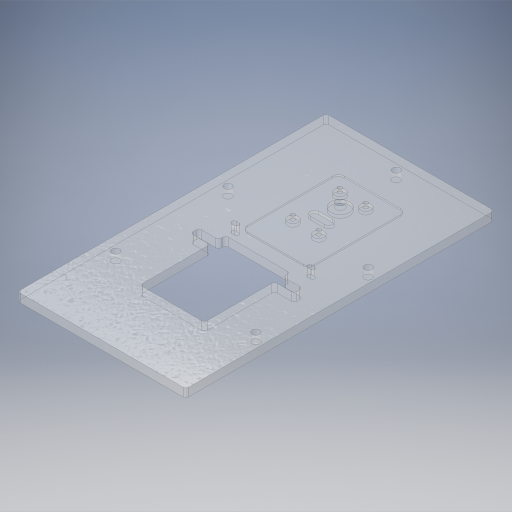
# Autodesk Inventor part: getriebe_platte_0
Saved by Autodesk Inventor 2023 (Build 270158000, 158)
## iProperties
Company: HTBLA Kaindorf
RuleStatus: InUse
Created: 2022-08-03
Part Number: getriebe_platte_0
Project: Zeichenmaschine_v2
Material: Acryl
Description: Platte Getriebemotor
Document SubType Name: Modeling
Designer: trajan20
Density: 1.188 g/cm^3
Appearance: Transparent - farblos
Mass: 160.681 g
Surface Area: 535.055 cm^2
Volume: 135.253 cm^3
AfterDocNew0: iProperties-Editor_aufrufen
Author: jan
Keywords: 2021
Autodesk Inventor part; units mm, degrees
ref_plane "YZ Plane" through (0, 0, 0) normal (1, 0, 0) x (0, 1, 0)
ref_plane "XZ Plane" through (0, 0, 0) normal (0, 1, 0) x (-1, 0, 0)
derived "BT000_trajan20_22_Zeichenmaschine_neu_Masterskizze.ipt"
sketch "Skizze3" plane through (0, 0, 0) normal (0, 0, 1) x (1, 0, 0)
  line L0 (0, 0) -> (-110, 0)
  line L1 (-220, 0) -> (-220, 120)
  line L2 (-220, 120) -> (0, 120)
  line L3 (0, 120) -> (0, 0)
  line L4 (-248.2253, 60) -> (-229.9902, 60) construction
  line L5 (-110, -37.5982) -> (-110, -22.8575) construction
  line L6 (-110, 0) -> (-220, 0)
  point P0 (-220, 60)
  point P1 (-110, 120)
  point P2 (-165, 0)
  point P3 (-60, 10)
  point P4 (-140, 10)
  point P5 (-140, 110)
  point P6 (-60, 110)
  point P7 (-60, 10)
  point P8 (-210, 60)
  dimension "d4" = 120
  dimension "d5" = 220
  dimension "d40" = 10
  dimension "d41" = 10
  dimension "d42" = 10
  dimension "d43" = 10
  dimension "d51" = 80
  dimension "d52" = 80
  dimension "d64" = 60
  dimension "d142" = 10
  dimension "d143" = 60
  constraints: 14 end point, 3 horizontal, 3 midpoint, 3 parallel, 3 point on line, 2 perpendicular, 1 coincident, 1 vertical, 1 vertical alignment
  measures "d4" distance between parallel lines of L0 L2
  measures "d5" distance between parallel lines of L1 L3
  measures "d40" distance from line of L2 point (-60, 110)
  measures "d41" distance from line of L0 point (-60, 10)
  measures "d42" distance from line of L6 point (-140, 10)
  measures "d43" distance from line of L2 point (-140, 110)
  measures "d51" distance from line of L1 point (-140, 10)
  measures "d52" distance from line of L1 point (-140, 110)
  measures "d64" distance from line of L3 point (-60, 10)
  measures "d142" distance from line of L1 point (-210, 60)
  measures "d143" distance from line of L6 point (-210, 60)
extrude "Extrusion3" add sketch "Skizze3" against normal blind 6
fillet "Rundung1" radius 2 4 edges at (-220, 120, -3) (-220, 0, -3) (0, 120, -3) (0, 0, -3)
hole "Bohrung2" at (-60, 10, 0) at (-140, 10, 0) at (-140, 110, 0) at (-60, 110, 0) at (-210, 60, 0) direction (0, 0, -1) diameter 5.5 end through all
derived "Getriebemotor.ipt"
ref_plane "Arbeitsebene3" through (0, 0, -4) normal (0, 0, -1) x (-1, 0, 0)
sketch "Skizze5" plane through (0, 0, -4) normal (0, 0, -1) x (-1, 0, 0)
  line L0 (138.8, 44) -> (138.8, 76)
  circle A0 centre (179.05, 69.25) radius 1.55
  circle A1 centre (179.05, 69.25) radius 3.775
  circle A2 centre (145.55, 69.25) radius 3.775
  circle A3 centre (145.55, 69.25) radius 1.55
  circle A4 centre (145.55, 50.75) radius 3.775
  circle A5 centre (145.55, 50.75) radius 1.55
  circle A6 centre (170, 60) radius 3.1
  circle A7 centre (170, 60) radius 6.675
  line L1 (184.8, 76) -> (184.8, 44)
  line L2 (184.8, 44) -> (138.8, 44)
  line L3 (138.8, 76) -> (184.8, 76)
  circle A8 centre (179.05, 50.75) radius 1.55
  circle A9 centre (179.05, 50.75) radius 3.775
  line L4 (220, 2) -> (220, 118) projected
  line L5 (218, 120) -> (2, 120) projected
  line L6 (0, 118) -> (0, 2) projected
  line L7 (156.8, 65) -> (156.8, 55) construction
  line L8 (153.7, 65) -> (153.7, 55)
  line L9 (159.9, 55) -> (159.9, 65)
  arc A10 (159.9, 65) -> (153.7, 65) centre (156.8, 65) ccw
  arc A11 (153.7, 55) -> (159.9, 55) centre (156.8, 55) ccw
  point P0 (0, 0)
  point P1 (184.8, 60)
  point P2 (220, 60)
  point P3 (138.8, 60)
  point P4 (0, 60)
  point P5 (156.8, 60)
  dimension "d112" = 6.75
  dimension "d113" = 6.75
  dimension "d114" = 6.75
  dimension "d115" = 6.75
  dimension "d116" = 32
  dimension "d117" = 46
  dimension "d124" = 3.1
  dimension "d125" = 3.1
  dimension "d126" = 7.55
  dimension "d127" = 16
  dimension "d128" = 14.8
  dimension "d129" = 5.75
  dimension "d131" = 5.75
  dimension "d132" = 6.75
  dimension "d133" = 6.75
  dimension "d135" = 13.35
  dimension "d136" = 3.1
  dimension "d137" = 7.55
  dimension "d138" = 7.55
  dimension "d139" = 3.1
  dimension "d140" = 50
  dimension "d242" = 6.2
  dimension "d243" = 18
  dimension "d244" = 10
  dimension "d245" = 6.2
  constraints: 16 end point, 12 centre point, 5 concentric, 5 midpoint, 5 parallel, 4 point on circle, 4 tangent, 3 horizontal alignment, 1 equal radius, 1 vertical
  measures "d112" distance from line of L2 A4.centre
  measures "d113" distance from line of L0 A4.centre
  measures "d114" distance from line of L0 A3.centre
  measures "d115" distance from line of L3 A3.centre
  measures "d116" distance of L0.start L0.end
  measures "d117" distance of L1.end L0.start
  measures "d124" diameter of A5
  measures "d125" diameter of A3
  measures "d126" diameter of A2
  measures "d127" distance from line of L2 A7.centre
  measures "d128" distance from line of L1 A7.centre
  measures "d129" distance from line of L1 A1.centre
  measures "d131" distance from line of L1 A8.centre
  measures "d132" distance from line of L2 A8.centre
  measures "d133" distance from line of L3 A0.centre
  measures "d135" diameter of A7
  measures "d136" diameter of A8
  measures "d137" diameter of A9
  measures "d138" diameter of A1
  measures "d139" diameter of A0
  measures "d140" distance from line of L4 A6.centre
  measures "d242" diameter of A6
  measures "d243" distance from line of L0 point (156.8, 60)
  measures "d244" distance of L7.start L7.end
  measures "d245" distance between parallel lines of L8 L9
sketch "Skizze6" plane through (0, 0, -6) normal (0, 0, -1) x (-1, 0, 0)
  circle A0 centre (60, 110) radius 2.75 projected
  circle A1 centre (140, 10) radius 2.75 projected
  circle A2 centre (60, 10) radius 2.75 projected
  circle A3 centre (140, 110) radius 2.75 projected
  circle A4 centre (210, 60) radius 2.75 projected
  arc A5 (0, 2) -> (2, 0) centre (2, 2) ccw projected
  line L0 (2, 0) -> (218, 0) projected
  arc A6 (218, 0) -> (220, 2) centre (218, 2) ccw projected
  line L1 (220, 2) -> (220, 118) projected
  arc A7 (220, 118) -> (218, 120) centre (218, 118) ccw projected
  line L2 (218, 120) -> (2, 120) projected
  arc A8 (2, 120) -> (0, 118) centre (2, 118) ccw projected
  line L3 (0, 118) -> (0, 2) projected
  circle A9 centre (179.05, 69.25) radius 3.775 projected
  line L4 (138.8, 76) -> (184.8, 76) projected
  line L5 (184.8, 76) -> (184.8, 44) projected
  circle A10 centre (179.05, 50.75) radius 3.775 projected
  circle A11 centre (179.05, 50.75) radius 1.55 projected
  line L6 (184.8, 44) -> (138.8, 44) projected
  line L7 (138.8, 44) -> (138.8, 76) projected
  circle A12 centre (145.55, 50.75) radius 3.775 projected
  circle A13 centre (145.55, 50.75) radius 1.55 projected
  circle A14 centre (145.55, 69.25) radius 3.775 projected
  circle A15 centre (145.55, 69.25) radius 1.55 projected
  circle A16 centre (170, 60) radius 6.675 projected
  circle A17 centre (170, 60) radius 3.1 projected
  circle A18 centre (179.05, 69.25) radius 1.55 projected
  line L8 (123.8, 84) -> (192.8, 84)
  line L9 (192.8, 84) -> (192.8, 36)
  line L10 (192.8, 36) -> (123.8, 36)
  line L11 (123.8, 36) -> (123.8, 84)
  line L12 (138.8, 62.5) -> (103.8, 62.5)
  line L13 (138.8, 57.5) -> (103.8, 57.5)
  line L14 (103.8, 67.5) -> (138.8, 67.5)
  line L15 (138.8, 57.5) -> (103.8, 67.5) construction
  line L16 (103.8, 57.5) -> (138.8, 67.5) construction
  line L17 (97.7, 99.5) -> (103.8, 99.5)
  line L18 (97.7, 25.5) -> (97.7, 99.5)
  line L19 (97.7, 85.5) -> (47.7, 85.5)
  line L20 (47.7, 39.5) -> (97.7, 39.5)
  line L21 (103.8, 99.5) -> (103.8, 25.5)
  line L22 (103.8, 25.5) -> (97.7, 25.5)
  line L23 (47.7, 39.5) -> (47.7, 85.5)
  line L24 (119.8, 90.5) -> (119.8, 88.5) construction
  line L25 (118.2, 90.5) -> (118.2, 88.5)
  line L26 (121.4, 88.5) -> (121.4, 90.5)
  arc A19 (121.4, 90.5) -> (118.2, 90.5) centre (119.8, 90.5) ccw
  arc A20 (118.2, 88.5) -> (121.4, 88.5) centre (119.8, 88.5) ccw
  line L27 (119.8, 36.5) -> (119.8, 34.5) construction
  line L28 (118.2, 36.5) -> (118.2, 34.5)
  line L29 (121.4, 34.5) -> (121.4, 36.5)
  arc A21 (121.4, 36.5) -> (118.2, 36.5) centre (119.8, 36.5) ccw
  arc A22 (118.2, 34.5) -> (121.4, 34.5) centre (119.8, 34.5) ccw
  line L30 (103.8, 39.5) -> (108.8, 39.5)
  line L31 (108.8, 39.5) -> (108.8, 85.5)
  line L32 (108.8, 85.5) -> (95.8, 85.5)
  line L33 (159.9, 55) -> (159.9, 65) projected
  line L34 (153.7, 65) -> (153.7, 55) projected
  arc A23 (159.9, 65) -> (153.7, 65) centre (156.8, 65) ccw projected
  arc A24 (153.7, 55) -> (159.9, 55) centre (156.8, 55) ccw projected
  point P0 (0, 0)
  point P1 (138.8, 60)
  point P2 (123.8, 60)
  point P3 (121.3, 62.5)
  point P4 (138.8, 67.5)
  point P5 (138.8, 57.5)
  point P6 (92.3, 62.6)
  point P7 (95.8, 62.6)
  point P8 (97.7, 62.5)
  point P9 (97.7, 39.5)
  point P10 (47.7, 62.5)
  point P11 (119.8, 89.5)
  point P12 (119.8, 35.5)
  point P13 (100.75, 25.5)
  point P14 (108.8, 67.5)
  point P15 (102.3, 85.5)
  point P16 (103.8, 85.5)
  dimension "d158" = 8
  dimension "d159" = 8
  dimension "d160" = 15
  dimension "d161" = 8
  dimension "d165" = 10
  dimension "d170" = 6.1
  dimension "d174" = 50
  dimension "d175" = 46
  dimension "d191" = 23
  dimension "d220" = 50
  dimension "d225" = 16
  dimension "d226" = 16
  dimension "d227" = 10
  dimension "d228" = 10
  dimension "d229" = 2
  dimension "d230" = 2
  dimension "d231" = 1.6
  dimension "d232" = 1.6
  dimension "d235" = 74
  dimension "d236" = 5
  dimension "d237" = 46
  dimension "d265" = 18.5
  dimension "d266" = 35
  dimension "d267" = 5
  constraints: 54 end point, 12 midpoint, 8 parallel, 8 point on circle, 8 tangent, 6 horizontal, 4 centre point, 4 point on line, 4 vertical, 3 perpendicular, 1 horizontal alignment
  measures "d158" distance between parallel lines of L4 L8
  measures "d159" distance between parallel lines of L6 L10
  measures "d160" distance of point (138.8, 60) point (123.8, 60)
  measures "d161" distance between parallel lines of L5 L9
  measures "d165" distance of L13.end L14.start
  measures "d170" distance of L17.start L17.end
  measures "d174" distance of L20.start L20.end
  measures "d175" distance of L19.end L20.start
  measures "d191" distance between parallel lines of L19 L12
  measures "d220" distance from line of L18 point (47.7, 62.5)
  measures "d225" distance from line of point (119.8, 35.5) L21
  measures "d226" distance from line of L21 point (119.8, 89.5)
  measures "d227" vertical distance of point (119.8, 35.5) point (100.75, 25.5)
  measures "d228" vertical distance of L17.end point (119.8, 89.5)
  measures "d229" distance of L27.start L27.end
  measures "d230" distance of L24.start L24.end
  measures "d231" radius of A19
  measures "d232" radius of A22
  measures "d235" distance from line of L21.end L17
  measures "d236" distance of L30.start L30.end
  measures "d237" distance of L30.end L31.end
  measures "d265" distance between parallel lines of L6 L12
  measures "d266" distance between parallel lines of L7 L21
  measures "d267" distance between parallel lines of L12 L13
extrude "Extrusion10" cut sketch "Skizze6" against normal blind 1 contours L7 L14 L11 L8 L9 L10 L13 L6 L5 L4 | L4 L5 L6 L7 | L7 L12 L11 L14 | L7 L13 L11 L12 | A24 L34 A23 L33
extrude "Extrusion11" cut sketch "Skizze6" against normal blind 3.2 contours A9 | A10 | A12 | A14 | A16 | A18 | A24 L34 A23 L33
extrude "Extrusion12" cut sketch "Skizze6" against normal blind 8 contours A11 | A13 | A15 | A17 | A18
fillet "Rundung3" radius 4 4 edges at (-123.8, 84, -5.5) (-192.8, 84, -5.5) (-192.8, 36, -5.5) (-123.8, 36, -5.5)
extrude "Extrusion13" cut sketch "Skizze6" against normal blind 8 contours L21 L22 L18 L32 | L32 L18 L17 L21 | L18 L20 L23 L19
fillet "Rundung4" radius 2 8 edges at (-97.7, 99.5, -3) (-103.8, 99.5, -3) (-97.7, 25.5, -3) (-97.7, 39.5, -3) (-97.7, 85.5, -3) (-47.7, 39.5, -3) (-47.7, 85.5, -3) (-103.8, 25.5, -3)
extrude "Extrusion14" cut sketch "Skizze6" against normal blind 8 contours A19 L26 A20 L25 | A21 L29 A22 L28
extrude "Extrusion15" cut sketch "Skizze6" against normal blind 10 contours L31 L12 L21 L14 | L14 L21 L32 L31 | L31 L13 L21 L12 | L31 L30 L21 L13
fillet "Rundung5" radius 2 4 edges at (-103.8, 39.5, -3) (-108.8, 39.5, -3) (-108.8, 85.5, -3) (-103.8, 85.5, -3)
equation "\"d4\" = Basis_Zubau_Breite_Profillänge + 4 * AluProfil_Abstand"
equation "\"d5\" = Basis_Zubau_Länge_Profillänge + 2 * AluProfil_Abstand"
equation "\"d41\" = d40"
equation "\"d42\" = d41"
equation "\"d43\" = d42"
equation "\"d127\" = 0.5 * d116"
equation "\"Basis_Zubau_Breite_Profillänge\" = 80"
equation "\"AluProfil_Abstand\" = 10"
equation "\"Basis_Zubau_Länge_Profillänge\" = 200"
